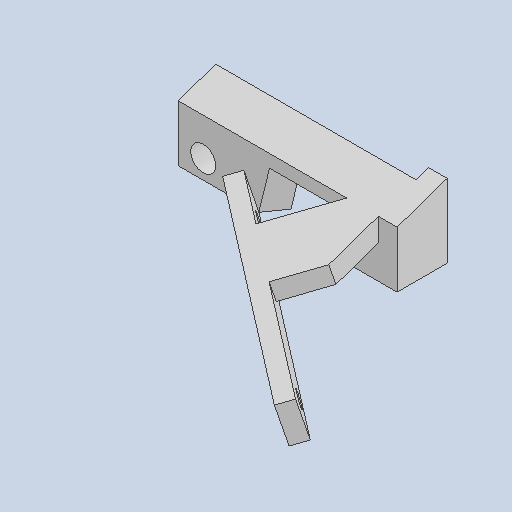
# Autodesk Inventor part: angle_09
Saved by Autodesk Inventor 2024.4 (Build 284460000, 460)
## iProperties
Created: 2026-04-06
Part Number: angle_09
Material: Generic
Document SubType Name: Modeling
Designer: tooles01
Density: 1 g/cm^3
Appearance: Default
Author: tooles01
Autodesk Inventor part; units mm, degrees
ref_plane "YZ Plane" through (0, 0, 0) normal (1, 0, 0) x (0, 1, 0)
ref_plane "XZ Plane" through (0, 0, 0) normal (0, 1, 0) x (-1, 0, 0)
ref_plane "XY Plane" through (0, 0, 0) normal (0, 0, 1) x (1, 0, 0)
sketch "Sketch: connect to post" plane through (0, 0, 0) normal (1, 0, 0) x (0, 1, 0)
  line L0 (11, 1) -> (2, 1)
  line L1 (2, 1) -> (2, -2)
  line L2 (2, -2) -> (10, -2)
  line L3 (11, -5) -> (11, 1)
  line L4 (10, -2) -> (10, -5)
  line L5 (10, -5) -> (11, -5)
  line L6 (9.5, -2.5) -> (-0.5, -2.5) construction
  line L7 (-0.5, -2.5) -> (-0.5, -12.5) construction
  line L8 (-0.5, -12.5) -> (9.5, -12.5) construction
  line L9 (9.5, -12.5) -> (9.5, -2.5) construction
  point P0 (0, 0)
  dimension "d129" = 10
  dimension "d130" = 1
  dimension "d132" = 8
  dimension "d148" = 3
  dimension "d159" = 3
  dimension "d162" = 0.5
  dimension "d163" = 0.5
  constraints: 20 end point, 9 perpendicular, 2 horizontal, 1 other
  measures "d129" distance of L7.end L8.end
  measures "d130" distance of L4.end L3.start
  measures "d132" distance of L1.end L2.end
  measures "d148" distance of L0.end L1.end
  measures "d159" distance of L2.end L4.end
  measures "d162" distance between parallel lines of L9 L4
  measures "d163" distance between parallel lines of L2 L6
sketch "Sketch1: angle down" plane through (0, 0, 0) normal (1, 0, 0) x (0, 1, 0)
  line L0 (11, 1) -> (5.7909, 16.1283)
  line L1 (5.7909, 16.1283) -> (2.4816, 14.9888)
  line L2 (2.4816, 14.9888) -> (7.6907, -0.1395)
  line L3 (7.6907, -0.1395) -> (11, 1)
  line L4 (0, -9.1875) -> (0, 20.1247) construction
  line L5 (11, 1) -> (2, 1) construction
  line L6 (11, -5) -> (11, 1) construction
  line L7 (2, 1) -> (2, -2) construction
  point P0 (0, 0)
  dimension "thickness" = 3.5
  dimension "d9" = 16
  dimension "angle_vertical" = 19
  constraints: 8 end point, 2 perpendicular, 1 parallel
  measures "thickness" distance of L0.end L1.end
  measures "d9" distance of L0.start L0.end
  measures "angle_vertical" angle of L4 L2
extrude "Ex1: down" add sketch "Sketch1: angle down" against normal blind 13
sketch "Sketch2: angle side" plane through (-13, 11.1299, 0.6227) normal (0, 0.9455186, 0.3255682) x (1, 0, 0)
  line L0 (7.2607, -16.399) -> (0, -10.9277)
  line L1 (0, -10.9277) -> (7.1196, -1.4797)
  line L2 (7.1196, -1.4797) -> (14.3803, -6.9511)
  line L3 (14.3803, -6.9511) -> (7.2607, -16.399)
  line L4 (7.1196, -1.4797) -> (12.9231, 6.2219)
  line L5 (13, -0.399) -> (13, -16.399) projected
  line L6 (13, -0.399) -> (0, -0.399) projected
  line L7 (0, -16.399) -> (0, -0.399) projected
  line L8 (13, -16.399) -> (0, -16.399) projected
  line L9 (0, -16.399) -> (0, -0.399) projected
  line L10 (14.3803, -6.9511) -> (15.2149, -5.8435)
  point P0 (10, -1.1071)
  point P1 (13, -8.7827)
  point P2 (0, -10.9277)
  point P3 (0, -10.9277)
  point P4 (6.4268, -0.399)
  point P5 (8.3395, -0.399)
  point P6 (13, -4.0451)
  point P7 (13, -5.9109)
  point P8 (7.9339, -0.399)
  dimension "d118" = 9.0914
  dimension "d119" = 11.8301
  dimension "angle_horizontal" = 37
  constraints: 12 end point, 2 collinear, 2 parallel, 2 point on line, 1 perpendicular
  measures "d118" distance of L0.start L0.end
  measures "d119" distance of L2.end L0.start
  measures "angle_horizontal" angle of L1 L7
extrude "Ex2: angle side" cut sketch "Sketch2: angle side" against normal up to surface (3.5 mm away) contours L8 L7 L0 | L3 L5 L8 | L7 L6 L4 L1
sketch "Sketch: mount to Arducam" plane through (-13, 7.5722, 10.955) normal (-0.601815, -0.2600103, 0.7551247) x (0.7986355, -0.1959318, 0.5690273)
  circle A0 centre (-4.4543, -4.5) radius 1.3
  circle A1 centre (23.5457, -4.5) radius 1.3
  line L0 (-8.4543, 0) -> (27.5457, 0)
  line L1 (27.5457, 0) -> (27.5457, -7.25)
  line L2 (27.5457, -7.25) -> (-8.4543, -7.25)
  line L3 (-8.4543, -7.25) -> (-8.4543, 0)
  line L4 (-4.4543, -4.5) -> (23.5457, -4.5) construction
  line L5 (24.6877, -7.16) -> (18.2457, -7.16)
  line L6 (18.2457, -7.16) -> (18.2457, -7.25)
  line L7 (24.6877, -7.25) -> (24.6877, -7.16)
  line L8 (0.9457, -7) -> (-2.0543, -7)
  line L9 (-2.0543, -7) -> (-2.0543, -7.25)
  line L10 (0.9457, -7.25) -> (0.9457, -7)
  line L11 (0, 0) -> (9.0914, 0) projected
  line L12 (9.0914, -3.5) -> (0, -3.5) projected
  line L13 (0.7257, -7.47) -> (-0.8543, -7.47) construction
  line L14 (-0.8543, -7.47) -> (-0.8543, -9.68) construction
  line L15 (-0.8543, -9.68) -> (0.7257, -9.68) construction
  line L16 (0.7257, -9.68) -> (0.7257, -7.47) construction
  line L17 (-1.9743, -9.2) -> (-4.9743, -9.2) construction
  line L18 (-4.9743, -9.2) -> (-4.9743, -11.7) construction
  line L19 (-4.9743, -11.7) -> (-1.9743, -11.7) construction
  line L20 (-1.9743, -11.7) -> (-1.9743, -9.2) construction
  line L21 (5.1957, -10.37) -> (-1.1743, -10.37) construction
  line L22 (-1.1743, -10.37) -> (-1.1743, -11.99) construction
  line L23 (-1.1743, -11.99) -> (5.1957, -11.99) construction
  line L24 (5.1957, -11.99) -> (5.1957, -10.37) construction
  line L25 (23.6297, -8.9) -> (21.1877, -8.9) construction
  line L26 (21.1877, -8.9) -> (21.1877, -11.18) construction
  line L27 (21.1877, -11.18) -> (23.6297, -11.18) construction
  line L28 (23.6297, -11.18) -> (23.6297, -8.9) construction
  line L29 (20.3957, -7.66) -> (18.8811, -7.66) construction
  line L30 (18.8811, -7.66) -> (18.8811, -8.45) construction
  line L31 (18.8811, -8.45) -> (20.3957, -8.45) construction
  line L32 (20.3957, -8.45) -> (20.3957, -7.66) construction
  point P0 (5.6322, -10.7263)
  point P1 (9.5457, -4.5)
  point P2 (9.5457, 0)
  point P3 (-8.02, -12.062)
  point P4 (-1.82, -12.062)
  point P5 (15.77, -12.062)
  point P6 (22.142, -12.062)
  point P7 (4.5457, 0)
  dimension "M2_throughhole" = 2.6
  dimension "d136" = 28
  dimension "d137" = 36
  dimension "d138" = 7.25
  dimension "d139" = 2.66
  dimension "d140" = 2.5
  dimension "d141" = 1.142
  dimension "d142" = 5.3
  dimension "d143" = 4.5
  dimension "d145" = 5.4
  dimension "d149" = 3
  dimension "d151" = 19
  dimension "d154" = 2.75
  dimension "d176" = 2.5
  dimension "d177" = 3
  dimension "d178" = 4.7
  dimension "d179" = 1.58
  dimension "d180" = 2.21
  dimension "d181" = 6.37
  dimension "d184" = 3.6
  dimension "d185" = 1.73
  dimension "d188" = 0.8
  dimension "d189" = 1.12
  dimension "d190" = 0.69
  dimension "d191" = 1.62
  dimension "d192" = 3.15
  dimension "d193" = 0.792
  dimension "d194" = 0.79
  dimension "d195" = 0.45
  dimension "d196" = 4.4
  constraints: 62 end point, 22 perpendicular, 9 horizontal, 4 point on line, 3 midpoint, 2 centre point, 2 coincident, 1 collinear, 1 equal radius, 1 vertical alignment
  measures "M2_throughhole" diameter of A0
  measures "d136" distance of L4.start L4.end
  measures "d137" distance of L0.start L0.end
  measures "d138" distance of L2.end L0.start
  measures "d139" distance from line of A1.centre L5
  measures "d140" distance from line of L8 L4.start
  measures "d141" distance from line of L7 A1.centre
  measures "d142" distance from line of L6 A1.centre
  measures "d143" distance between parallel lines of L0 L4
  measures "d145" distance from line of A0.centre L10
  measures "d149" distance of L8.start L8.end
  measures "d151" horizontal distance of A1.centre point (4.546, 0)
  measures "d154" distance from line of L2 A0.centre
  measures "d176" distance of L17.end L18.end
  measures "d177" distance of L18.end L19.end
  measures "d178" distance from line of L17 L4.start
  measures "d179" distance of L13.start L13.end
  measures "d180" distance of L15.end L13.start
  measures "d181" distance of L22.end L23.end
  measures "d184" distance from line of L4.start L14
  measures "d185" distance between parallel lines of L13 L17
  measures "d188" distance between parallel lines of L20 L22
  measures "d189" distance between parallel lines of L14 L20
  measures "d190" distance between parallel lines of L21 L15
  measures "d191" distance of L23.end L21.start
  measures "d192" distance from line of L32 A1.centre
  measures "d193" distance between parallel lines of L32 L26
  measures "d194" distance of L29.end L30.end
  measures "d195" distance between parallel lines of L25 L31
  measures "d196" distance from line of L25 A1.centre
extrude "Ex5: mount to Arducam" add sketch "Sketch: mount to Arducam" against normal blind 2.5
extrude "Ex1: connect to post" add sketch "Sketch: connect to post" against normal blind 32
sketch "Sketch: hole for screw into post" plane through (0, 2, 1) normal (0, 0, 1) x (1, 0, 0)
  circle A0 centre (-28, 3) radius 2
  line L0 (0, 8) -> (-32, 8) construction
  line L1 (-32, 0) -> (-32, 9) construction
  point P0 (0, -2)
  dimension "d127" = 5
  dimension "d128" = 4
  dimension "d133" = 4
  constraints: 1 centre point
  measures "d127" distance from line of A0.centre L0
  measures "d128" diameter of A0
  measures "d133" distance from line of A0.centre L1
extrude "Ex1a: hole for screw into post" cut sketch "Sketch: hole for screw into post" against normal blind 20
sketch "Sketch: for printing" plane through (0, 0, 0) normal (1, 0, 0) x (0, 1, 0)
  line L0 (11, -5) -> (12.7348, -4.0384)
  line L1 (12.7348, -4.0384) -> (11, 1)
  line L2 (11, -5) -> (11, 1) projected
  line L3 (11, 1) -> (2, 1) projected
  line L4 (11, -5) -> (13.066, -5)
  line L5 (13.066, -5) -> (12.7348, -4.0384)
  line L6 (11, -5) -> (11, 1) projected
  point P0 (0, 0)
  dimension "d156" = 19
  dimension "d161" = 80
  constraints: 8 end point, 1 collinear, 1 perpendicular
  measures "d156" angle of L2 L1
  measures "d161" angle of L1 L0
extrude "Ex: for printing" add sketch "Sketch: for printing" against normal up to surface (32 mm away)
sketch "Sketch: access camera nut" plane through (-11.4955, 8.2222, 9.0672) normal (0.601815, 0.2600103, -0.7551247) x (-0.7986355, 0.1959318, -0.5690273)
  circle A0 centre (4.4543, -4.5) radius 1.3 construction
  line L0 (0.9543, -1.9222) -> (9.4543, -1.9222)
  line L1 (9.4543, -1.9222) -> (9.4543, -9.4864)
  line L2 (9.4543, -9.4864) -> (0.9543, -9.4864)
  line L3 (0.9543, -9.4864) -> (0.9543, -1.9222)
  line L4 (-4.1023, -9.4864) -> (21.4541, -9.4864) projected
  line L5 (-2.5348, -1.9222) -> (23.0215, -1.9222) projected
  dimension "d168" = 3.5
  dimension "d170" = 5
  constraints: 8 end point, 3 perpendicular, 2 collinear
  measures "d168" distance from line of L3 A0.centre
  measures "d170" distance from line of L1 A0.centre
extrude "Ex: access camera nut" cut sketch "Sketch: access camera nut" along normal up to surface surface through (0, 10, -2) normal (0, 0, -1)
sketch "Sketch: text" plane through (-5.9742, 7.2983, 1) normal (0, -0.9455186, -0.3255682) x (1, 0, 0)
  line L0 (-3.1439, 6.5064) -> (6.9988, 6.5064) construction
  line L1 (6.9988, 6.5064) -> (6.9988, -0.4772) construction
  line L2 (6.9988, -0.4772) -> (-3.1439, -0.4772) construction
  line L3 (-3.1439, -0.4772) -> (-3.1439, 6.5064) construction
  line L4 (-1.6375, 5.336) -> (-0.4826, 5.336)
  line L5 (-0.4826, 5.336) -> (0.0834, 3.4996)
  line L6 (0.0834, 3.4996) -> (0.6647, 5.336)
  line L7 (0.6647, 5.336) -> (1.785, 5.336)
  line L8 (1.785, 5.336) -> (0.5531, 2.4371)
  line L9 (0.5531, 2.4371) -> (-0.4325, 2.4371)
  line L10 (-0.4325, 2.4371) -> (-1.6375, 5.336)
  line L11 (2.0468, 3.3341) -> (3.1517, 3.4727)
  spline S0 degree 2 poles (3.1517, 3.4727) (3.1941, 3.2417) (3.4019, 3.0492) (3.5521, 3.0492) knots 0 0 0 1 2 2 2
  spline S1 degree 2 poles (3.5521, 3.0492) (3.8216, 3.0492) (3.9717, 3.3187) knots 0 0 0 1 1 1
  spline S2 degree 2 poles (3.9717, 3.3187) (4.0795, 3.5189) (4.1334, 4.1656) knots 0 0 0 1 1 1
  spline S3 degree 2 poles (4.1334, 4.1656) (3.9332, 3.9616) (3.5136, 3.7691) (3.2403, 3.7691) knots 0 0 0 1 2 2 2
  spline S4 degree 2 poles (3.2403, 3.7691) (2.7013, 3.7691) (1.9621, 4.5314) (1.9621, 5.1166) knots 0 0 0 1 2 2 2
  spline S5 degree 2 poles (1.9621, 5.1166) (1.9621, 5.5169) (2.3394, 6.1714) (2.9977, 6.5064) (3.4982, 6.5064) knots 0 0 0 1 2 3 3 3
  spline S6 degree 2 poles (3.4982, 6.5064) (4.0988, 6.5064) (4.8225, 6.0944) (5.2576, 5.1974) (5.2576, 4.4582) knots 0 0 0 1 2 3 3 3
  spline S7 degree 2 poles (5.2576, 4.4582) (5.2576, 3.3764) (4.3452, 2.3678) (3.5405, 2.3678) knots 0 0 0 1 2 2 2
  spline S8 degree 2 poles (3.5405, 2.3678) (3.0632, 2.3678) (2.5088, 2.5872) (2.1469, 3.0145) (2.0468, 3.3341) knots 0 0 0 1 2 3 3 3
  spline S9 degree 2 poles (4.0911, 5.1204) (4.0911, 5.4438) (3.7638, 5.8134) (3.529, 5.8134) knots 0 0 0 1 2 2 2
  spline S10 degree 2 poles (3.529, 5.8134) (3.3095, 5.8134) (3.017, 5.4823) (3.017, 5.1474) knots 0 0 0 1 2 2 2
  spline S11 degree 2 poles (3.017, 5.1474) (3.017, 4.8124) (3.3211, 4.4582) (3.5482, 4.4582) knots 0 0 0 1 2 2 2
  spline S12 degree 2 poles (3.5482, 4.4582) (3.7831, 4.4582) (4.0911, 4.8009) (4.0911, 5.1204) knots 0 0 0 1 2 2 2
  point P0 (5.9742, 1.4306)
  constraints: 2 other
extrude "Ex: text" cut sketch "Sketch: text" against normal blind 1
sketch "Sketch: end cap" plane through (0, 0, 0) normal (1, 0, 0) x (0, 0, -1)
  line L0 (5, 13.066) -> (-8.927, 8.2705) projected
  line L1 (5, 10) -> (5, 13.066) projected
  line L2 (2, 10) -> (5, 10) projected
  line L3 (2, 2) -> (2, 10) projected
  line L4 (-1, 2) -> (2, 2) projected
  line L5 (-1, 7.2983) -> (-1, 2) projected
  line L6 (-1, 11) -> (-1, 7.2983)
  line L7 (5, 13.066) -> (7, 13.7546)
  line L8 (7, 13.7546) -> (7, 2)
  line L9 (7, 2) -> (2, 2)
  point P0 (0, 0)
  dimension "d173" = 5
  constraints: 8 end point, 3 collinear, 1 perpendicular, 1 point on line
  measures "d173" distance of L8.end L3.start
extrude "Ex: end cap" add sketch "Sketch: end cap" along normal blind 3
body "Solid1"
